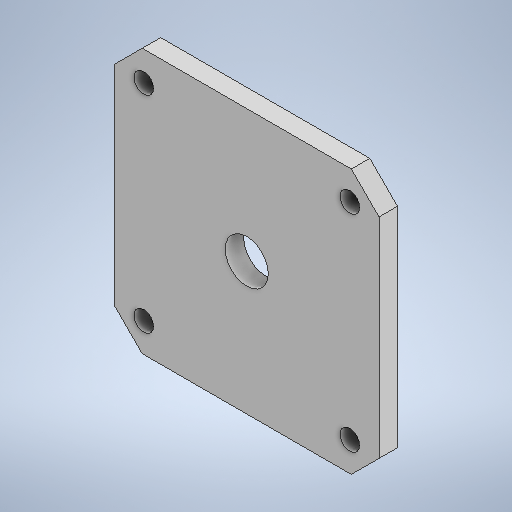
# Autodesk Inventor part: DC Motor Fixation
Saved by Autodesk Inventor 2025.4 (Build 294407000, 407)
## iProperties
Created: 2026-05-07
Part Number: DC Motor Fixation
Material: Generic
Document SubType Name: Sheet Metal
Designer: lenovo
Density: 1 g/cm^3
Sheet Metal Rule: Default_mm
Appearance: Default
Author: lenovo
Autodesk Inventor part; units mm, degrees
ref_plane "YZ Plane" through (0, 0, 0) normal (1, 0, 0) x (0, 1, 0)
ref_plane "XZ Plane" through (0, 0, 0) normal (0, 1, 0) x (-1, 0, 0)
ref_plane "XY Plane" through (0, 0, 0) normal (0, 0, 1) x (1, 0, 0)
sketch "Sketch1" plane through (0, 0, 0) normal (0, 0, 1) x (1, 0, 0)
  line L0 (-21.5, -21.5) -> (21.5, -21.5)
  line L1 (21.5, -21.5) -> (21.5, 21.5)
  line L2 (21.5, 21.5) -> (-21.5, 21.5)
  line L3 (-21.5, 21.5) -> (-21.5, -21.5)
  line L4 (-21.5, -21.5) -> (21.5, 21.5) construction
  line L5 (21.5, -21.5) -> (-21.5, 21.5) construction
  point P0 (0, 0)
  dimension "d0" = 43
  dimension "d1" = 43
  measures "d0" distance of L2.end L1.end
  measures "d1" distance of L1.end L0.end
extrude "Plate1" add sketch "Sketch1" along normal blind 3
chamfer "Corner Chamfer1" distance 4.5 angle 45 4 edges at (21.5, 21.5, 1.5) (-21.5, 21.5, 1.5) (-21.5, -21.5, 1.5) (21.5, -21.5, 1.5)
sketch "Sketch2" plane through (0, 0, 3) normal (0, 0, 1) x (1, 0, 0)
  line L0 (-17, 21.5) -> (17, 21.5) projected
  line L1 (0, 21.5) -> (0, -21.5)
  line L2 (17, -21.5) -> (-17, -21.5) projected
  line L3 (-21.5, -17) -> (-21.5, 17) projected
  line L4 (-21.5, 0) -> (21.5, 0)
  line L5 (21.5, 17) -> (21.5, -17) projected
  circle A0 centre (-16.75, 16.75) radius 1.6
  circle A1 centre (16.75, 16.75) radius 1.6
  circle A2 centre (-16.75, -16.75) radius 1.6
  circle A3 centre (16.75, -16.75) radius 1.6
  circle A4 centre (0, 0) radius 3.5
  dimension "d6" = 3.2
  dimension "d7" = 33.5
  dimension "d8" = 33.5
  dimension "d11" = 7
  constraints: 5 centre point, 4 end point, 4 midpoint, 3 symmetric about line, 1 coincident, 3 other
  measures "d6" diameter of A0
  measures "d7" diameter of A0.centre L1
  measures "d8" diameter of A0.centre L4
  measures "d11" diameter of A4
extrude "Cut1" cut sketch "Sketch2" against normal blind 3
equation "\"d9\" = Thickness"
equation "\"d2\" = Thickness"
equation "\"BendRadius\" = Thickness"
equation "\"BendReliefWidth\" = Thickness"
equation "\"BendReliefDepth\" = 0.5 * Thickness"
equation "\"CornerReliefSize\" = 4 * Thickness"
equation "\"MinimumRemnant\" = 2 * Thickness"
equation "\"TransitionRadius\" = BendRadius"
equation "\"JacobiRadiusSize\" = BendRadius"
equation "\"GapSize\" = Thickness"
equation "\"Thickness\" = 3"
body "Solid1"
